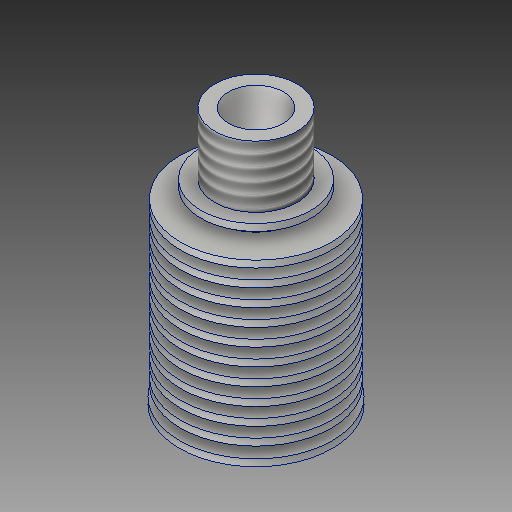
# Autodesk Inventor part: Threaded Heatsink
Saved by Autodesk Inventor 2019 (Build 230136000, 136)
## iProperties
Created: 2018-10-01
Part Number: Threaded Heatsink
Material: Aluminum 6061
Document SubType Name: Modeling
Designer: Ax
Density: 2.7 g/cm^3
Appearance: Aluminum - Flat
Author: Ax
Autodesk Inventor part; units mm, degrees
ref_plane "YZ Plane" through (0, 0, 0) normal (1, 0, 0) x (0, 1, 0)
ref_plane "XZ Plane" through (0, 0, 0) normal (0, 1, 0) x (-1, 0, 0)
ref_plane "XY Plane" through (0, 0, 0) normal (0, 0, 1) x (1, 0, 0)
sketch "Sketch1" plane through (0, 0, 0) normal (0, 0, 1) x (1, 0, 0)
  line L0 (-11, -11.75) -> (-11, -10.75)
  line L1 (-11, -10.75) -> (-6, -10.75)
  line L2 (-6, -10.75) -> (-6, -9.25)
  line L3 (-6, -9.25) -> (-11, -9.25)
  line L4 (-11, -9.25) -> (-11, -8.25)
  line L5 (-11, -8.25) -> (-6, -8.25)
  line L6 (-6, -8.25) -> (-6, -6.75)
  line L7 (-6, -6.75) -> (-11, -6.75)
  line L8 (-11, -6.75) -> (-11, -5.75)
  line L9 (-11, -5.75) -> (-6, -5.75)
  line L10 (-6, -5.75) -> (-6, -4.25)
  line L11 (-6, -4.25) -> (-11, -4.25)
  line L12 (-11, -4.25) -> (-11, -3.25)
  line L13 (-11, -3.25) -> (-6, -3.25)
  line L14 (-6, -3.25) -> (-6, -1.75)
  line L15 (-6, -1.75) -> (-11, -1.75)
  line L16 (-11, -1.75) -> (-11, -0.75)
  line L17 (-11, -0.75) -> (-6, -0.75)
  line L18 (-6, -0.75) -> (-6, 0.75)
  line L19 (-6, 0.75) -> (-11, 0.75)
  line L20 (-11, 0.75) -> (-11, 1.75)
  line L21 (-11, 1.75) -> (-6, 1.75)
  line L22 (-6, 1.75) -> (-6, 3.25)
  line L23 (-6, 3.25) -> (-11, 3.25)
  line L24 (-11, 3.25) -> (-11, 4.25)
  line L25 (-11, 4.25) -> (-6, 4.25)
  line L26 (-6, 4.25) -> (-6, 5.75)
  line L27 (-6, 5.75) -> (-11, 5.75)
  line L28 (-11, 5.75) -> (-11, 6.75)
  line L29 (-11, 6.75) -> (-6, 6.75)
  line L30 (-6, 6.75) -> (-6, 8.25)
  line L31 (-6, 8.25) -> (-11, 8.25)
  line L32 (-11, 8.25) -> (-11, 9.25)
  line L33 (-11, 9.25) -> (-6, 9.25)
  line L34 (-6, 9.25) -> (-6, 10.75)
  line L35 (-6, 10.75) -> (-11, 10.75)
  line L36 (-11, 10.75) -> (-11, 11.75)
  line L37 (-11, 11.75) -> (-6, 11.75)
  line L38 (-6, 11.75) -> (-6, 13.25)
  line L39 (-11, -11.75) -> (-6, -11.75)
  line L40 (0, 0) -> (0, 10.5257) construction
  line L41 (0, 0) -> (-17.6287, 0) construction
  line L42 (-11.15, -13.25) -> (-11.15, -14.25)
  line L43 (-11.15, -14.25) -> (-3, -14.25)
  line L44 (-3, -14.25) -> (-3, 0.85)
  line L45 (-3, 0.85) -> (-2.1, 2)
  line L46 (-2.1, 2) -> (-2.1, 23.25)
  line L47 (-6, 13.25) -> (-8, 13.25)
  line L48 (-8, 13.25) -> (-8, 14.25)
  line L49 (-8, 14.25) -> (-6, 14.25)
  line L50 (-6, 14.25) -> (-6, 23.25)
  line L51 (-6, 23.25) -> (-2.1, 23.25)
  line L52 (-11.15, -13.25) -> (-6, -13.25)
  line L53 (-6, -13.25) -> (-6, -11.75)
  line L54 (0, -21.75) -> (0, 30.75) projected
  dimension "d5" = 1
  dimension "d6" = 1.5
  dimension "d7" = 11
  dimension "d8" = 11.15
  dimension "d9" = 3
  dimension "d10" = 15.1
  dimension "d11" = 2.1
  dimension "d12" = 37.5
  dimension "d13" = 26
  dimension "d14" = 28.5
  dimension "d16" = 8
  dimension "d17" = 6
  dimension "d18" = 21.25
  constraints: 108 end point, 28 equal length, 25 perpendicular, 18 point on line, 15 vertical, 10 horizontal, 1 parallel, 1 symmetric about line
  measures "d5" distance of L3.end L4.end
  measures "d6" distance of L1.end L2.end
  measures "d7" distance from line of L0 L40.start
  measures "d8" horizontal distance of L40.start L42.end
  measures "d9" horizontal distance of L40.start L43.end
  measures "d10" distance of L43.end L44.end
  measures "d11" horizontal distance of L40.start L45.end
  measures "d12" vertical distance of L46.end L43.end
  measures "d13" vertical distance of L36.end L42.end
  measures "d14" distance from line of L48.end L43
  measures "d16" horizontal distance of L47.end L40.start
  measures "d17" horizontal distance of L40.start L50.end
  measures "d18" distance of L45.end L46.end
revolve "Revolution1" add sketch "Sketch1" angle 360 about axis through (0, -10, 0) along (0, 1, 0)
thread "Thread1" size "M12x1.75" class "6g" standard "ISO Metric profile" full length
sketch "Sketch2" plane through (0, 23.25, 0) normal (0, 1, 0) x (1, 0, 0)
  circle A0 centre (0, 0) radius 4
  dimension "d22" = 8
  constraints: 1 centre point, 1 coincident
  measures "d22" diameter of A0
extrude "Extrusion1" cut sketch "Sketch2" against normal blind 6
body "Solid1"
